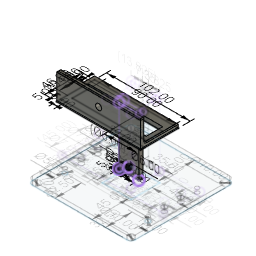
assembly (Autodesk Fusion 360 design; units mm, degrees)
Autodesk Fusion 360 part; units mm, degrees
sketch "Sketch1" plane through (0, 0, 0) normal (0, 0, 1) x (1, 0, 0) in component "Main plate"
  line L0 (5, 0) -> (120, 0)
  line L1 (125, 5) -> (125, 120)
  line L2 (120, 125) -> (5, 125)
  line L3 (0, 120) -> (0, 5)
  arc A0 (125, 120) -> (120, 125) centre (120, 120) ccw
  arc A1 (5, 125) -> (0, 120) centre (5, 120) ccw
  arc A2 (0, 5) -> (5, 0) centre (5, 5) ccw
  arc A3 (120, 0) -> (125, 5) centre (120, 5) ccw
  circle A4 centre (12, 32.5) radius 2.5
  circle A5 centre (113, 32.5) radius 2.5
  circle A6 centre (12, 92.5) radius 2.5
  line L4 (45, 80) -> (80, 80)
  line L5 (80, 80) -> (80, 45)
  line L6 (80, 45) -> (45, 45)
  line L7 (45, 45) -> (45, 80)
  dimension "d3" = 10
  dimension "d4" = 10
  dimension "d5" = 10
  dimension "d6" = 10
  dimension "d7" = 5
  dimension "d8" = 12
  dimension "d9" = 32.5
  dimension "d10" = 5
  dimension "d11" = 12
  dimension "d12" = 32.5
  dimension "d13" = 5
  dimension "d15" = 12
  dimension "d16" = 32.5
  dimension "d81" = 35
  dimension "d82" = 35
  dimension "d83" = 45
  dimension "d84" = 45
  dimension "d85" = 45
  dimension "d86" = 45
  constraint horizontal L0
  constraint vertical L1
  constraint horizontal L2
  constraint vertical L3
  constraint tangent L2 A0
  constraint tangent L1 A0
  constraint tangent L2 A1
  constraint tangent L3 A1
  constraint tangent L3 A2
  constraint tangent L0 A2
  constraint tangent L1 A3
  constraint tangent L0 A3
  constraint horizontal L4
  constraint vertical L5
  constraint horizontal L6
  constraint vertical L7
  measures "d3" diameter of A0
  measures "d4" diameter of A1
  measures "d5" diameter of A2
  measures "d6" diameter of A3
  measures "d7" diameter of A4
  measures "d8" distance of L3 A4.centre
  measures "d9" distance of L0 A4.centre
  measures "d10" diameter of A5
  measures "d11" distance of L1 A5.centre
  measures "d12" distance of L0 A5.centre
  measures "d13" diameter of A6
  measures "d15" distance of L3 A6.centre
  measures "d16" distance of L2 A6.centre
  measures "d81" distance of L4.start L4.end
  measures "d82" distance of L4.start L6.end
  measures "d83" distance of L0 L6
  measures "d84" distance of L3 L7
  measures "d85" distance of L1 L5
  measures "d86" distance of L2 L4
extrude "Extrude1" add sketch "Sketch1" along normal blind 5 contours L0 L1 L2 L3 A0 A1 A2 A3 | L4 L5 L6 L7 makes body 1 in component "Main plate"
sketch "Sketch1 (2)" plane through (0, 0, 0) normal (0, 0, 1) x (1, 0, 0) in component "Holder"
  line L0 (0, 0) -> (125, 0)
  line L1 (125, 0) -> (125, 25)
  line L2 (125, 25) -> (0, 25)
  line L3 (0, 25) -> (0, 0)
  circle A0 centre (12, 8) radius 2.55
  circle A1 centre (113, 8) radius 2.55
  line L4 (23.5147, 12.5) -> (94.9191, 12.5) construction
  line L5 (0, 20) -> (125, 20)
  dimension "d21" = 125
  dimension "d22" = 25
  dimension "d23" = 5.1
  dimension "d24" = 5.1
  dimension "d25" = 8
  dimension "d26" = 8
  dimension "d27" = 12
  dimension "d28" = 12
  dimension "d29" = 12.5
  dimension "d30" = 5
  constraint horizontal L0
  constraint vertical L1
  constraint horizontal L2
  constraint vertical L3
  constraint coincident L0.start L3.end
  constraint horizontal L4
  constraint coincident L3 L5.start
  constraint coincident L1 L5.end
  constraint perpendicular L1 L5
  measures "d21" distance of L0.start L0.end
  measures "d22" distance of L0.start L2.end
  measures "d23" diameter of A0
  measures "d24" diameter of A1
  measures "d25" distance of L0 A0.centre
  measures "d26" distance of L0 A1.centre
  measures "d27" distance of L3 A0.centre
  measures "d28" distance of L1 A1.centre
  measures "d29" distance of L0 L4
  measures "d30" distance of L2 L5
extrude "Extrude1'" add sketch "Sketch1 (2)" along normal blind 5 separate body contours L0 L1 L3 L5 makes body 2 in component "Holder"
extrude "Extrude2" add sketch "Sketch1 (2)" along normal blind 100 contours L1 L2 L3 L5 bodies 2 in component "Holder"
fillet "Fillet1" radius 3 1 edges at (62.5, 20, 5) on bodies 2 in component "Holder"
sketch "Sketch2" plane through (0, 20, 0) normal (0, -1, 0) x (1, 0, 0) in component "Holder"
sketch "Sketch3" plane through (0, 20, 0) normal (0, -1, 0) x (1, 0, 0) in component "Holder"
  line L0 (125, 100) -> (0, 100)
  line L1 (62.5, 100) -> (62.5, 8) construction
  line L2 (125, 8) -> (125, 100)
  line L3 (125, 8) -> (0, 8)
  circle A0 centre (62.5, 94.325) radius 3.675
  circle A1 centre (62.5, 82.975) radius 3.675
  circle A2 centre (62.5, 84.175) radius 3.275
  circle A3 centre (62.5, 84.175) radius 3.275
  circle A4 centre (62.5, 73.625) radius 3.275
  circle A5 centre (62.5, 63.075) radius 3.275
  circle A6 centre (62.5, 52.525) radius 3.275
  circle A7 centre (62.5, 52.525) radius 3.275
  circle A8 centre (62.5, 41.975) radius 3.275
  circle A9 centre (62.5, 31.425) radius 3.275
  circle A10 centre (62.5, 20.875) radius 3.275
  dimension "d37" = 62.5
  dimension "cam_diameter" = 7.35
  dimension "d39" = 5.675
  dimension "d40" = 7.35
  dimension "d41" = 11.35
  dimension "d42" = 6.55
  dimension "d43" = 6.55
  dimension "d44" = 6.55
  dimension "d45" = 6.55
  dimension "d46" = 6.55
  dimension "d47" = 6.55
  dimension "d48" = 6.55
  dimension "d49" = 6.55
  dimension "d50" = 6.55
  constraint perpendicular L0 L1
  constraint midpoint L0 L1.start
  constraint midpoint L1.end L3
  constraint coincident L1 A0.centre
  measures "d37" distance of L1 L2
  measures "cam_diameter" diameter of A0
  measures "d39" distance of L1.start A0.centre
  measures "d40" diameter of A1
  measures "d41" distance of A0.centre A1.centre
  measures "d42" diameter of A2
  measures "d43" diameter of A3
  measures "d44" diameter of A4
  measures "d45" diameter of A5
  measures "d46" diameter of A6
  measures "d47" diameter of A7
  measures "d48" diameter of A8
  measures "d49" diameter of A9
  measures "d50" diameter of A10
extrude "Extrude3" cut sketch "Sketch3" against normal blind 5 bodies 2 in component "Holder"
fillet "Fillet2" radius 1 15 edges at (0, 22.5, 100) (62.5, 25, 100) (125, 22.5, 100) (125, 8.5, 5) (125, 19.1213, 5.8787) (125, 20, 54) (125, 25, 50) (125, 12.5, 0) (62.5, 0, 5) (62.5, 0, 0) (0, 20, 54) (0, 19.1213, 5.8787) (0, 8.5, 5) (0, 12.5, 0) (0, 25, 50) on bodies 2 in component "Holder"
sketch "Sketch4" plane through (0, 20, 0) normal (0, -1, 0) x (1, 0, 0) in component "Holder"
  line L0 (11, 90) -> (52.5, 90)
  line L1 (52.5, 90) -> (52.5, 18)
  line L2 (52.5, 18) -> (11, 18)
  line L3 (11, 18) -> (11, 90)
  line L4 (1, 8) -> (1, 100)
  line L5 (125, 100) -> (0, 100)
  line L6 (125, 8) -> (0, 8)
  line L7 (72.5, 90) -> (114, 90)
  line L8 (114, 90) -> (114, 18)
  line L9 (114, 18) -> (72.5, 18)
  line L10 (72.5, 18) -> (72.5, 90)
  point P0 (62.5, 73.625)
  point P1 (62.5, 82.975)
  dimension "d55" = 10
  dimension "d56" = 10
  dimension "d57" = 10
  dimension "d58" = 10
  dimension "d59" = 72
  dimension "d60" = 41.5
  dimension "d61" = 41.5
  dimension "d62" = 72
  dimension "d63" = 10
  dimension "d64" = 10
  constraint horizontal L0
  constraint vertical L1
  constraint horizontal L2
  constraint vertical L3
  constraint horizontal L7
  constraint vertical L8
  constraint horizontal L9
  constraint vertical L10
  measures "d55" distance of L3 L4
  measures "d56" distance of L1 P0
  measures "d57" distance of L0 L5
  measures "d58" distance of L2 L6
  measures "d59" distance of L0.start L2.end
  measures "d60" distance of L0.start L0.end
  measures "d61" distance of L7.start L7.end
  measures "d62" distance of L7.start L9.end
  measures "d63" distance of L10 P1
  measures "d64" distance of L6 L9
sketch "Sketch2 (2)" plane through (0, 0, 5) normal (0, 0, 1) x (-1, 0, 0) in component "Main plate"
  circle A0 centre (-12, -72.5) radius 3
  line L0 (0, -120) -> (0, -5)
  circle A1 centre (-12, -52.5) radius 3
  circle A2 centre (-113, -52.5) radius 3
  line L1 (-125, -5) -> (-125, -120)
  circle A3 centre (-113, -72.5) radius 3
  circle A4 centre (-113, -92.5) radius 2.5
  line L2 (-120, -125) -> (-5, -125)
  point P0 (-12, -92.5)
  point P1 (-12, -32.5)
  point P2 (-113, -32.5)
  dimension "d65" = 6
  dimension "d66" = 20
  dimension "d67" = 12
  dimension "d68" = 6
  dimension "d69" = 20
  dimension "d70" = 12
  dimension "d71" = 20
  dimension "d72" = 6
  dimension "d73" = 12
  dimension "d74" = 6
  dimension "d75" = 12
  dimension "d148" = 5
  dimension "d149" = 20
  dimension "d150" = 20
  dimension "d151" = 20
  dimension "d152" = 32.5
  dimension "d153" = 12
  measures "d65" diameter of A0
  measures "d66" vertical distance of A0.centre P0
  measures "d67" distance of A0.centre L0
  measures "d68" diameter of A1
  measures "d69" vertical distance of A0.centre A1.centre
  measures "d70" distance of L0 A1.centre
  measures "d71" distance of A1.centre P1
  measures "d72" diameter of A2
  measures "d73" distance of A2.centre L1
  measures "d74" diameter of A3
  measures "d75" distance of L1 A3.centre
  measures "d148" diameter of A4
  measures "d149" vertical distance of A3.centre A4.centre
  measures "d150" distance of A2.centre A3.centre
  measures "d151" vertical distance of A2.centre P2
  measures "d152" distance of A4.centre L2
  measures "d153" distance of L1 A4.centre
sketch "Sketch3 (2)" plane through (0, 0, 5) normal (0, 0, 1) x (-1, 0, 0) in component "Main plate"
extrude "Extrude2'" add sketch "Sketch2 (2)" against normal blind 5 contours A0 | A1 | A2 | A3 bodies 1 in component "Main plate"
extrude "Extrude3'" cut sketch "Sketch2 (2)" against normal blind 5 contours A0 | A1 | A2 | A3 bodies 1 in component "Main plate"
sketch "Sketch1 (3)" plane through (0, 0, 0) normal (0, 0, 1) x (1, 0, 0) in component "slider"
  line L0 (0, 0) -> (-123, 0)
  line L1 (-123, 0) -> (-123, 45)
  line L2 (-123, 45) -> (0, 45)
  line L3 (0, 45) -> (0, 0)
  circle A0 centre (-112, 32.5) radius 3.5
  circle A1 centre (-112, 12.5) radius 3.5
  circle A2 centre (-11, 32.5) radius 3.5
  circle A3 centre (-11, 12.5) radius 3.5
  dimension "slider_lower_width" = 123
  dimension "slider_lower_height" = 45
  dimension "d90" = 7
  dimension "d91" = 7
  dimension "d92" = 7
  dimension "d93" = 7
  dimension "d97" = 12.5
  dimension "d98" = 12.5
  dimension "d99" = 11
  dimension "d100" = 11
  dimension "d101" = 11
  dimension "d102" = 12.5
  dimension "d103" = 11
  dimension "d104" = 12.5
  constraint horizontal L0
  constraint vertical L1
  constraint horizontal L2
  constraint vertical L3
  constraint coincident L0.start L3.end
  measures "slider_lower_width" distance of L0.start L0.end
  measures "slider_lower_height" distance of L0.start L2.end
  measures "d90" diameter of A0
  measures "d91" diameter of A1
  measures "d92" diameter of A2
  measures "d93" diameter of A3
  measures "d97" distance of L2 A0.centre
  measures "d98" distance of L0 A1.centre
  measures "d99" distance of L1 A1.centre
  measures "d100" distance of L1 A0.centre
  measures "d101" distance of L3 A3.centre
  measures "d102" distance of L0 A3.centre
  measures "d103" distance of L3 A2.centre
  measures "d104" distance of L2 A2.centre
extrude "Extrude1''" add sketch "Sketch1 (3)" along normal blind 5 separate body makes body 3 in component "slider"
fillet "Fillet1'" radius 2 1 edges at (0, 0, 2.5) on bodies 3 in component "slider"
fillet "Fillet2'" radius 2 1 edges at (0, 45, 2.5) on bodies 3 in component "slider"
fillet "Fillet3" radius 2 1 edges at (-123, 45, 2.5) on bodies 3 in component "slider"
fillet "Fillet4" radius 2 1 edges at (-123, 0, 2.5) on bodies 3 in component "slider"
sketch "Sketch2 (3)" plane through (0, 0, 5) normal (0, 0, 1) x (-1, 0, 0) in component "slider"
  point P0 (112, -32.5)
  point P1 (11, -32.5)
  dimension "d115" = 101
  measures "d115" distance of P0 P1
sketch "Sketch3 (3)" plane through (0, 0, 5) normal (0, 0, 1) x (-1, 0, 0) in component "slider"
  line L0 (79, -5) -> (79, -40)
  line L1 (79, -40) -> (44, -40)
  line L2 (44, -40) -> (44, -5)
  line L3 (0, 0) -> (123, 0)
  line L4 (123, 0) -> (123, -45)
  line L5 (0, -45) -> (0, 0)
  line L6 (74, -5) -> (74, -35)
  line L7 (74, -35) -> (49, -35)
  line L8 (49, -35) -> (49, -5)
  line L9 (44, -5) -> (49, -5)
  line L10 (74, -5) -> (79, -5)
  point P0 (112, -12.5)
  point P1 (11, -12.5)
  dimension "d116" = 35
  dimension "d117" = 35
  dimension "d118" = 5
  dimension "d119" = 44
  dimension "d120" = 44
  dimension "d121" = 33
  dimension "d122" = 33
  dimension "d123" = 5
  dimension "d124" = 5
  dimension "d125" = 5
  constraint horizontal L9
  constraint vertical L0
  constraint horizontal L1
  constraint vertical L2
  constraint coincident L6.start L9
  constraint perpendicular L6 L9
  constraint perpendicular L6 L7
  constraint perpendicular L8 L9
  constraint collinear L9 L10
  measures "d116" distance of L2.end L0.start
  measures "d117" distance of L2.end L1.end
  measures "d118" distance of L3 L9
  measures "d119" distance of L0 L4
  measures "d120" distance of L2 L5
  measures "d121" distance of L0 P0
  measures "d122" distance of L2 P1
  measures "d123" distance of L0 L6
  measures "d124" distance of L2 L8
  measures "d125" distance of L1 L7
extrude "Extrude2''" add sketch "Sketch3 (3)" along normal blind 80 bodies 3 in component "slider"
fillet "Fillet5" radius 2 3 edges at (-79, 22.5, 5) (-61.5, 40, 5) (-44, 22.5, 5) on bodies 3 in component "slider"
fillet "Fillet6" radius 2 8 edges at (-0.5858, 0.5858, 5) (0, 22.5, 5) (-0.5858, 44.4142, 5) (-61.5, 45, 5) (-122.4142, 44.4142, 5) (-123, 22.5, 5) (-122.4142, 0.5858, 5) (-61.5, 0, 5) on bodies 3 in component "slider"
fillet "Fillet7" radius 2 2 edges at (-45.5, 5, 5) (-77.5, 5, 5) on bodies 3 in component "slider"
sketch "Sketch4 (2)" plane through (0, 0, 85) normal (0, 0, 1) x (-1, 0, 0) in component "slider"
  line L0 (49, -35) -> (49, -5)
  line L1 (74, -5) -> (74, -35)
  dimension "d134" = 25
  measures "d134" distance of L0 L1
sketch "Sketch5" plane through (0, 40, 0) normal (0, 1, 0) x (-1, 0, 0) in component "slider"
sketch "Sketch6" plane through (0, 0, 85) normal (0, 0, 1) x (-1, 0, 0) in component "slider"
sketch "Sketch7" plane through (0, 0, 85) normal (0, 0, 1) x (-1, 0, 0) in component "slider"
sketch "Sketch8" plane through (0, 40, 0) normal (0, 1, 0) x (-1, 0, 0) in component "slider"
  line L0 (74, 85) -> (49, 85)
  line L1 (79, 7) -> (44, 7)
  line L2 (57.825, 85) -> (57.825, 7)
  line L3 (65.175, 7) -> (65.175, 85)
  line L4 (44, 7) -> (44, 85)
  line L5 (79, 7) -> (79, 85)
  dimension "d135" = 13.825
  dimension "d136" = 7.35
  dimension "d137" = 13.825
  constraint coincident L0 L2.start
  constraint coincident L1 L2.end
  constraint perpendicular L1 L2
  constraint coincident L1 L3.start
  constraint coincident L0 L3.end
  constraint perpendicular L0 L3
  measures "d135" distance of L2 L4
  measures "d136" distance of L2 L3
  measures "d137" distance of L3 L5
extrude "Extrude3''" cut sketch "Sketch8" against normal blind 5 bodies 3 in component "slider"
sketch "Sketch9" plane through (0, 0, 5) normal (0, 0, 1) x (-1, 0, 0) in component "slider"
  line L0 (123, -45) -> (0, -45)
  line L1 (0, 0) -> (123, 0)
  dimension "d140" = 45
  measures "d140" distance of L0 L1
sketch "Sketch4 (3)" plane through (0, 0, 5) normal (0, 0, 1) x (-1, 0, 0) in component "Main plate"
  circle A0 centre (-113, -92.5) radius 2.5
  line L0 (-120, -125) -> (-5, -125)
  line L1 (-125, -5) -> (-125, -120)
  dimension "d145" = 5
  dimension "d146" = 32.5
  dimension "d147" = 12
  measures "d145" diameter of A0
  measures "d146" distance of A0.centre L0
  measures "d147" distance of A0.centre L1
extrude "Extrude4" cut sketch "Sketch4 (3)" against normal blind 5 bodies 1 in component "Main plate"
sketch "Sketch10" plane through (-44, 0, 0) normal (1, 0, 0) x (0, 1, 0) in component "slider"
  line L0 (35, 85) -> (5, 85)
  line L1 (40, 7) -> (5, 7)
  dimension "d156" = 78
  measures "d156" distance of L0 L1
sketch "Sketch1 (4)" plane through (0, 0, 0) normal (0, 0, 1) x (1, 0, 0) in component "camera_holder"
sketch "Sketch2 (4)" plane through (0, 0, 0) normal (0, 0, 1) x (1, 0, 0) in component "camera_holder"
  line L0 (0, 0) -> (24, 0)
  line L1 (24, 0) -> (24, 5)
  line L2 (24, 5) -> (0, 5)
  line L3 (0, 5) -> (0, 0)
  dimension "d157" = 24
  dimension "d158" = 5
  constraint horizontal L0
  constraint vertical L1
  constraint horizontal L2
  constraint vertical L3
  constraint coincident L0.start L3.end
  measures "d157" distance of L0.start L0.end
  measures "d158" distance of L0.start L2.end
extrude "Extrude1'''" add sketch "Sketch2 (4)" along normal blind 70 separate body makes body 4 in component "camera_holder"
sketch "Sketch3 (4)" plane through (0, 0, 0) normal (0, -1, 0) x (1, 0, 0) in component "camera_holder"
  circle A0 centre (12, 8) radius 3
  line L0 (0, 0) -> (24, 0)
  line L1 (0, 0) -> (0, 70)
  dimension "d161" = 6
  dimension "d162" = 8
  dimension "d163" = 12
  measures "d161" diameter of A0
  measures "d162" distance of A0.centre L0
  measures "d163" distance of A0.centre L1
extrude "Extrude2'''" cut sketch "Sketch3 (4)" against normal blind 5 bodies 4 in component "camera_holder"
sketch "Sketch4 (4)" plane through (0, 0, 0) normal (0, -1, 0) x (1, 0, 0) in component "camera_holder"
sketch "Sketch5 (2)" plane through (0, 0, 0) normal (0, -1, 0) x (1, 0, 0) in component "camera_holder"
  circle A0 centre (12, 8) radius 3
  dimension "d166" = 6
  measures "d166" diameter of A0
sketch "Sketch6 (2)" plane through (0, 0, 70) normal (0, 0, 1) x (-1, 0, 0) in component "camera_holder"
  line L0 (39, -9) -> (-63, -9)
  line L1 (-63, -9) -> (-63, 37)
  line L2 (-63, 37) -> (39, 37)
  line L3 (39, 37) -> (39, -9)
  line L4 (-24, 0) -> (-24, -5)
  line L5 (-24, -5) -> (0, -5)
  line L6 (33, 4) -> (-57, 4)
  line L7 (-57, 4) -> (-57, 24)
  line L8 (-57, 24) -> (33, 24)
  line L9 (33, 24) -> (33, 4)
  line L10 (0, 0) -> (-24, 0)
  line L11 (39, 32) -> (-63, 32)
  dimension "d167" = 102
  dimension "d168" = 46
  dimension "d169" = 39
  dimension "d170" = 4
  dimension "d171" = 90
  dimension "d172" = 20
  dimension "d173" = 4
  dimension "d174" = 6
  dimension "d175" = 5
  constraint horizontal L0
  constraint vertical L1
  constraint horizontal L2
  constraint vertical L3
  constraint horizontal L6
  constraint vertical L7
  constraint horizontal L8
  constraint vertical L9
  constraint coincident L3 L11.start
  constraint coincident L1 L11.end
  constraint perpendicular L1 L11
  measures "d167" distance of L0.start L0.end
  measures "d168" distance of L0.start L2.end
  measures "d169" distance of L1 L4
  measures "d170" distance of L0 L5
  measures "d171" distance of L6.start L6.end
  measures "d172" distance of L6.start L8.end
  measures "d173" distance of L6 L10
  measures "d174" distance of L3 L9
  measures "d175" distance of L2 L11
extrude "Extrude3'''" add sketch "Sketch6 (2)" along normal blind 5 contours L0 L1 L3 L11 bodies 4 in component "camera_holder"
extrude "Extrude4'" add sketch "Sketch6 (2)" along normal blind 32 contours L1 L2 L3 L11 bodies 4 in component "camera_holder"
fillet "Fillet1''" radius 2 1 edges at (12, -32, 75) on bodies 4 in component "camera_holder"
fillet "Fillet2''" radius 1 14 edges at (12, -37, 102) (12, -32, 102) (63, -34.5, 102) (-39, -34.5, 102) (-39, -10.5, 75) (-39, -31.4142, 75.5858) (-39, -32, 89.5) (12, -37, 70) (63, -14, 70) (12, 9, 70) (12, 9, 75) (63, -32, 89.5) (63, -31.4142, 75.5858) (63, -10.5, 75) on bodies 4 in component "camera_holder"
sketch "Sketch7 (2)" plane through (0, -32, 0) normal (0, 1, 0) x (-1, 0, 0) in component "camera_holder"
  circle A0 centre (-12, 89.7801) radius 3.675
  line L0 (39, 77) -> (39, 101)
  dimension "d184" = 7.35
  dimension "d185" = 51
  measures "d184" diameter of A0
  measures "d185" distance of A0.centre L0
extrude "Extrude5" cut sketch "Sketch7 (2)" against normal blind 5 bodies 4 in component "camera_holder"
component "Main plate" placed x (1, 0, 0) y (0, 1, 0) z (0, 0, 1) at (-124, -40, -5)
component "slider" placed x (1, 0, 0) y (0, 1, 0) z (0, 0, 1) at (0, 0, 0)
component "camera_holder" placed x (1, 0, 0) y (0, 1, 0) z (0, 0, 1) at (-73.5, 20, 5)
equation "main_plate_thickness = 5 mm"
equation "d29 = d22 / 2"
equation "d31 = 5 mm"
equation "d37 = d21 / 2"
equation "d39 = cam_diameter / 2 + 2 mm"
equation "d41 = cam_diameter + 4 mm"
equation "d51 = -d31"
equation "d77 = -main_plate_thickness"
equation "d79 = -main_plate_thickness"
equation "upper_plate_thickness_1 = 5 mm"
equation "d163 = d157 / 2"
